Autodesk Fusion 360 part; units mm, degrees
(part 2 of 3)
  line L860 (200.8112, -803.4113) -> (192.1466, -803.4586)
  line L861 (192.1466, -803.4586) -> (192.1301, -800.4585)
  line L862 (192.1301, -800.4585) -> (183.5876, -800.5058)
  line L863 (183.5876, -800.5058) -> (183.6041, -803.5055)
  line L864 (183.6041, -803.5055) -> (174.9396, -803.5538)
  line L865 (174.9396, -803.5538) -> (174.923, -800.5538)
  line L866 (174.923, -800.5538) -> (166.3802, -800.6007)
  line L867 (166.3802, -800.6007) -> (166.3967, -803.6004)
  line L868 (166.3967, -803.6004) -> (157.7322, -803.6483)
  line L869 (157.7322, -803.6483) -> (157.7156, -800.6487)
  line L870 (157.7156, -800.6487) -> (149.1731, -800.6953)
  line L871 (149.1731, -800.6953) -> (149.1897, -803.6949)
  line L872 (149.1897, -803.6949) -> (140.5251, -803.7432)
  line L873 (140.5251, -803.7432) -> (137.5251, -803.7598)
  line L874 (137.5251, -803.7598) -> (137.5086, -800.7598)
  line L875 (137.5086, -800.7598) -> (137.5082, -800.6988)
  line L876 (137.5082, -800.6988) -> (140.5082, -800.6822)
  line L877 (140.5082, -800.6822) -> (140.5086, -800.7432)
  line L878 (140.5086, -800.7432) -> (140.4662, -793.059)
  line L879 (140.4662, -793.059) -> (137.4662, -793.0756)
  line L880 (137.4662, -793.0756) -> (137.4239, -785.3308)
  line L881 (137.4239, -785.3308) -> (140.4235, -785.3138)
  line L882 (140.4235, -785.3138) -> (140.3812, -777.691)
  line L883 (140.3812, -777.691) -> (137.3816, -777.7073)
  line L884 (137.3816, -777.7073) -> (137.3389, -769.9624)
  line L885 (137.3389, -769.9624) -> (140.3389, -769.9455)
  line L886 (140.3389, -769.9455) -> (140.2969, -762.323)
  line L887 (140.2969, -762.323) -> (137.2969, -762.3396)
  line L888 (137.2969, -762.3396) -> (137.2546, -754.5944)
  line L889 (137.2546, -754.5944) -> (140.2542, -754.5774)
  line L890 (140.2542, -754.5774) -> (140.2119, -746.9546)
  line L891 (140.2119, -746.9546) -> (137.2122, -746.9712)
  line L892 (137.2122, -746.9712) -> (137.1695, -739.226)
  line L893 (137.1695, -739.226) -> (140.1695, -739.2091)
  line L894 (140.1695, -739.2091) -> (140.1276, -731.5866)
  line L895 (140.1276, -731.5866) -> (137.1276, -731.6032)
  line L896 (137.1276, -731.6032) -> (137.0849, -723.858)
  line L897 (137.0849, -723.858) -> (140.0849, -723.8414)
  line L898 (140.0849, -723.8414) -> (140.0425, -716.2182)
  line L899 (140.0425, -716.2182) -> (137.0429, -716.2348)
  line L900 (137.0429, -716.2348) -> (137.0002, -708.49)
  line L901 (137.0002, -708.49) -> (140.0002, -708.473)
  line L902 (140.0002, -708.473) -> (139.9582, -700.8502)
  line L903 (139.9582, -700.8502) -> (136.9582, -700.8668)
  line L904 (136.9582, -700.8668) -> (136.9155, -693.1219)
  line L905 (136.9155, -693.1219) -> (139.9156, -693.105)
  line L906 (139.9156, -693.105) -> (139.8732, -685.4822)
  line L907 (139.8732, -685.4822) -> (136.8736, -685.4984)
  line L908 (136.8736, -685.4984) -> (136.8309, -677.7536)
  line L909 (136.8309, -677.7536) -> (139.8309, -677.7366)
  line L910 (139.8309, -677.7366) -> (139.7889, -670.1138)
  line L911 (139.7889, -670.1138) -> (136.7889, -670.1304)
  line L912 (136.7889, -670.1304) -> (136.7462, -662.3855)
  line L913 (136.7462, -662.3855) -> (139.7462, -662.3686)
  line L914 (139.7462, -662.3686) -> (139.7039, -654.6851)
  line L915 (139.7039, -654.6851) -> (139.7039, -654.7458)
  line L916 (139.7039, -654.7458) -> (136.7042, -654.762)
  line L917 (136.7042, -654.762) -> (136.7039, -654.7017)
  line L918 (136.7039, -654.7017) -> (136.6873, -651.7017)
  line L919 (136.6873, -651.7017) -> (139.6873, -651.6851)
  line L920 (139.6873, -651.6851) -> (148.3519, -651.6371)
  line L921 (148.3519, -651.6371) -> (148.3684, -654.6371)
  line L922 (148.3684, -654.6371) -> (156.9113, -654.5899)
  line L923 (156.9113, -654.5899) -> (156.8947, -651.5899)
  line L924 (156.8947, -651.5899) -> (165.5593, -651.5422)
  line L925 (165.5593, -651.5422) -> (165.5758, -654.5423)
  line L926 (165.5758, -654.5423) -> (174.1183, -654.4953)
  line L927 (174.1183, -654.4953) -> (174.1017, -651.4953)
  line L928 (174.1017, -651.4953) -> (182.7667, -651.4477)
  line L929 (182.7667, -651.4477) -> (182.7829, -654.4477)
  line L930 (182.7829, -654.4477) -> (191.3257, -654.4004)
  line L931 (191.3257, -654.4004) -> (191.3091, -651.4004)
  line L932 (191.3091, -651.4004) -> (199.9737, -651.3528)
  line L933 (199.9737, -651.3528) -> (199.9903, -654.3528)
  line L934 (199.9903, -654.3528) -> (208.5328, -654.3055)
  line L935 (208.5328, -654.3055) -> (208.5162, -651.3059)
  line L936 (208.5162, -651.3059) -> (217.1807, -651.2579)
  line L937 (217.1807, -651.2579) -> (217.1973, -654.2579)
  line L938 (217.1973, -654.2579) -> (225.7402, -654.211)
  line L939 (225.7402, -654.211) -> (225.7236, -651.211)
  line L940 (225.7236, -651.211) -> (234.3881, -651.163)
  line L941 (234.3881, -651.163) -> (234.4047, -654.163)
  line L942 (234.4047, -654.163) -> (242.9472, -654.1161)
  line L943 (242.9472, -654.1161) -> (242.931, -651.1161)
  line L944 (242.931, -651.1161) -> (251.5955, -651.0685)
  line L945 (251.5955, -651.0685) -> (251.6118, -654.0685)
  line L946 (251.6118, -654.0685) -> (260.1546, -654.0212)
  line L947 (260.1546, -654.0212) -> (260.138, -651.0212)
  line L948 (260.138, -651.0212) -> (268.8026, -650.9736)
  line L949 (268.8026, -650.9736) -> (268.8192, -653.9736)
  line L950 (268.8192, -653.9736) -> (277.362, -653.9263)
  line L951 (277.362, -653.9263) -> (277.3454, -650.9263)
  line L952 (277.3454, -650.9263) -> (286.01, -650.879)
  line L953 (286.01, -650.879) -> (286.0266, -653.879)
  line L954 (286.0266, -653.879) -> (294.5691, -653.8318)
  line L955 (294.5691, -653.8318) -> (294.5525, -650.8317)
  line L956 (294.5525, -650.8317) -> (303.217, -650.7841)
  line L957 (303.217, -650.7841) -> (303.2336, -653.7841)
  line L958 (303.2336, -653.7841) -> (311.7761, -653.7369)
  line L959 (311.7761, -653.7369) -> (311.7595, -650.7368)
  line L960 (311.7595, -650.7368) -> (320.4244, -650.6892)
  line L961 (320.4244, -650.6892) -> (320.441, -653.6889)
  line L962 (320.441, -653.6889) -> (328.9835, -653.6423)
  line L963 (328.9835, -653.6423) -> (328.9669, -650.6423)
  line L964 (328.9669, -650.6423) -> (337.6315, -650.5943)
  line L965 (337.6315, -650.5943) -> (337.6481, -653.5943)
  line L966 (337.6481, -653.5943) -> (346.1909, -653.5474)
  line L967 (346.1909, -653.5474) -> (346.1743, -650.5474)
  line L968 (346.1743, -650.5474) -> (354.8389, -650.4994)
  line L969 (354.8389, -650.4994) -> (354.8555, -653.4994)
  line L970 (354.8555, -653.4994) -> (363.3979, -653.4525)
  line L971 (363.3979, -653.4525) -> (363.3817, -650.4525)
  line L972 (363.3817, -650.4525) -> (372.0463, -650.4049)
  line L973 (372.0463, -650.4049) -> (372.0625, -653.4049)
  line L974 (372.0625, -653.4049) -> (380.6053, -653.3576)
  line L975 (380.6053, -653.3576) -> (380.5888, -650.3576)
  line L976 (380.5888, -650.3576) -> (389.2533, -650.31)
  line L977 (389.2533, -650.31) -> (389.2695, -653.31)
  line L978 (389.2695, -653.31) -> (397.8124, -653.2627)
  line L979 (397.8124, -653.2627) -> (397.7958, -650.2631)
  line L980 (397.7958, -650.2631) -> (406.4607, -650.2154)
  line L981 (406.4607, -650.2154) -> (406.4773, -653.2155)
  line L982 (406.4773, -653.2155) -> (415.0198, -653.1682)
  line L983 (415.0198, -653.1682) -> (415.0032, -650.1682)
  line L984 (415.0032, -650.1682) -> (423.6678, -650.1202)
  line L985 (423.6678, -650.1202) -> (423.6843, -653.1202)
  line L986 (423.6843, -653.1202) -> (432.2272, -653.0733)
  line L987 (432.2272, -653.0733) -> (432.2106, -650.0733)
  line L988 (432.2106, -650.0733) -> (440.8752, -650.0256)
  line L989 (440.8752, -650.0256) -> (440.8914, -653.0257)
  line L990 (440.8914, -653.0257) -> (449.4342, -652.9787)
  line L991 (449.4342, -652.9787) -> (449.4177, -649.9787)
  line L992 (449.4177, -649.9787) -> (458.0822, -649.9308)
  line L993 (458.0822, -649.9308) -> (458.0988, -652.9308)
  line L994 (458.0988, -652.9308) -> (466.6416, -652.8838)
  line L995 (466.6416, -652.8838) -> (466.6251, -649.8838)
  line L996 (466.6251, -649.8838) -> (475.2893, -649.8362)
  line L997 (475.2893, -649.8362) -> (475.3058, -652.8359)
  line L998 (475.3058, -652.8359) -> (483.8487, -652.789)
  line L999 (483.8487, -652.789) -> (483.8321, -649.7889)
  line L1000 (483.8321, -649.7889) -> (492.497, -649.7413)
  line L1001 (492.497, -649.7413) -> (492.5132, -652.7413)
  line L1002 (492.5132, -652.7413) -> (501.0557, -652.6941)
  line L1003 (501.0557, -652.6941) -> (501.0391, -649.694)
  line L1004 (501.0391, -649.694) -> (509.7041, -649.6464)
  line L1005 (509.7041, -649.6464) -> (509.7206, -652.6464)
  line L1006 (509.7206, -652.6464) -> (518.2635, -652.5995)
  line L1007 (518.2635, -652.5995) -> (518.2469, -649.5995)
  line L1008 (518.2469, -649.5995) -> (526.9111, -649.5515)
  line L1009 (526.9111, -649.5515) -> (526.9277, -652.5515)
  line L1010 (526.9277, -652.5515) -> (535.4705, -652.5046)
  line L1011 (535.4705, -652.5046) -> (535.4539, -649.5046)
  line L1012 (535.4539, -649.5046) -> (544.1185, -649.4566)
  line L1013 (544.1185, -649.4566) -> (544.1351, -652.4566)
  line L1014 (544.1351, -652.4566) -> (552.6776, -652.4097)
  line L1015 (552.6776, -652.4097) -> (552.6613, -649.4101)
  line L1016 (552.6613, -649.4101) -> (561.3255, -649.3621)
  line L1017 (561.3255, -649.3621) -> (561.3421, -652.3621)
  line L1018 (561.3421, -652.3621) -> (569.885, -652.3152)
  line L1019 (569.885, -652.3152) -> (569.8684, -649.3152)
  line L1020 (569.8684, -649.3152) -> (578.5329, -649.2672)
  line L1021 (578.5329, -649.2672) -> (578.5495, -652.2672)
  line L1022 (578.5495, -652.2672) -> (587.092, -652.2199)
  line L1023 (587.092, -652.2199) -> (587.0754, -649.2199)
  line L1024 (587.0754, -649.2199) -> (595.7403, -649.1726)
  line L1025 (595.7403, -649.1726) -> (598.7404, -649.1561)
  line L1026 (598.7404, -649.1561) -> (598.7569, -652.1561)
  line L1027 (598.7569, -652.1561) -> (598.7573, -652.2171)
  line L1028 (598.7573, -652.2171) -> (595.7573, -652.2333)
  line L1029 (3.1447, -620.2227) -> (3.1447, -628.8876)
  line L1030 (3.1447, -628.8876) -> (6.1443, -628.8876)
  line L1031 (6.1443, -620.2227) -> (3.1447, -620.2227)
  line L1032 (3.1447, -603.0153) -> (3.1447, -611.6799)
  line L1033 (3.1447, -611.6799) -> (6.1443, -611.6799)
  line L1034 (6.1443, -603.0153) -> (3.1447, -603.0153)
  line L1035 (3.1447, -585.8079) -> (3.1447, -594.4725)
  line L1036 (3.1447, -594.4725) -> (6.1443, -594.4725)
  line L1037 (6.1443, -585.8079) -> (3.1447, -585.8079)
  line L1038 (3.1447, -568.6002) -> (3.1447, -577.2651)
  line L1039 (3.1447, -577.2651) -> (6.1443, -577.2651)
  line L1040 (6.1443, -568.6002) -> (3.1447, -568.6002)
  line L1041 (3.1447, -551.3928) -> (3.1447, -560.0573)
  line L1042 (3.1447, -560.0573) -> (6.1443, -560.0573)
  line L1043 (6.1443, -551.3928) -> (3.1447, -551.3928)
  line L1044 (3.1447, -534.185) -> (3.1447, -542.8499)
  line L1045 (3.1447, -542.8499) -> (6.1443, -542.8499)
  line L1046 (6.1443, -534.185) -> (3.1447, -534.185)
  line L1047 (3.1447, -516.9776) -> (3.1447, -525.6425)
  line L1048 (3.1447, -525.6425) -> (6.1443, -525.6425)
  line L1049 (6.1443, -516.9776) -> (3.1447, -516.9776)
  line L1050 (3.1447, -499.7702) -> (3.1447, -508.4348)
  line L1051 (3.1447, -508.4348) -> (6.1443, -508.4348)
  line L1052 (6.1443, -499.7702) -> (3.1447, -499.7702)
  line L1053 (3.1447, -482.5625) -> (3.1447, -491.2274)
  line L1054 (3.1447, -491.2274) -> (6.1443, -491.2274)
  line L1055 (6.1443, -482.5625) -> (3.1447, -482.5625)
  line L1056 (3.1447, -465.3551) -> (3.1447, -474.02)
  line L1057 (3.1447, -474.02) -> (6.1443, -474.02)
  line L1058 (6.1443, -465.3551) -> (3.1447, -465.3551)
  line L1059 (3.1447, -448.1477) -> (3.1447, -456.8122)
  line L1060 (3.1447, -456.8122) -> (6.1443, -456.8122)
  line L1061 (6.1443, -448.1477) -> (3.1447, -448.1477)
  line L1062 (3.1447, -430.9403) -> (3.1447, -439.6048)
  line L1063 (3.1447, -439.6048) -> (6.1443, -439.6048)
  line L1064 (6.1443, -430.9403) -> (3.1447, -430.9403)
  line L1065 (3.1447, -413.7329) -> (3.1447, -422.3974)
  line L1066 (3.1447, -422.3974) -> (6.1443, -422.3974)
  line L1067 (6.1443, -413.7329) -> (3.1447, -413.7329)
  line L1068 (3.1447, -396.5255) -> (3.1447, -405.1897)
  line L1069 (3.1447, -405.1897) -> (6.1443, -405.1897)
  line L1070 (6.1443, -396.5255) -> (3.1447, -396.5255)
  line L1071 (3.1447, -379.3177) -> (3.1447, -387.9826)
  line L1072 (3.1447, -387.9826) -> (6.1443, -387.9826)
  line L1073 (6.1443, -379.3177) -> (3.1447, -379.3177)
  line L1074 (3.1447, -362.1103) -> (3.1447, -370.7752)
  line L1075 (3.1447, -370.7752) -> (6.1443, -370.7752)
  line L1076 (6.1443, -362.1103) -> (3.1447, -362.1103)
  line L1077 (3.1447, -344.9029) -> (3.1447, -353.5675)
  line L1078 (3.1447, -353.5675) -> (6.1443, -353.5675)
  line L1079 (6.1443, -344.9029) -> (3.1447, -344.9029)
  line L1080 (3.1447, -327.6952) -> (3.1447, -336.3601)
  line L1081 (3.1447, -336.3601) -> (6.1443, -336.3601)
  line L1082 (6.1443, -327.6952) -> (3.1447, -327.6952)
  line L1083 (3.1447, -310.4878) -> (3.1447, -319.1527)
  line L1084 (3.1447, -319.1527) -> (6.1443, -319.1527)
  line L1085 (6.1443, -310.4878) -> (3.1447, -310.4878)
  line L1086 (3.1447, -293.2804) -> (3.1447, -301.9449)
  line L1087 (3.1447, -301.9449) -> (6.1443, -301.9449)
  line L1088 (6.1443, -293.2804) -> (3.1447, -293.2804)
  line L1089 (3.1447, -276.0726) -> (3.1447, -284.7375)
  line L1090 (3.1447, -284.7375) -> (6.1443, -284.7375)
  line L1091 (6.1443, -276.0726) -> (3.1447, -276.0726)
  line L1092 (3.1447, -258.8652) -> (3.1447, -267.5298)
  line L1093 (3.1447, -267.5298) -> (6.1443, -267.5298)
  line L1094 (6.1443, -258.8652) -> (3.1447, -258.8652)
  line L1095 (3.1447, -241.6578) -> (3.1447, -250.3224)
  line L1096 (3.1447, -250.3224) -> (6.1443, -250.3224)
  line L1097 (6.1443, -241.6578) -> (3.1447, -241.6578)
  line L1098 (3.1447, -224.4501) -> (3.1447, -233.115)
  line L1099 (3.1447, -233.115) -> (6.1443, -233.115)
  line L1100 (6.1443, -224.4501) -> (3.1447, -224.4501)
  line L1101 (3.1447, -207.2427) -> (3.1447, -215.9072)
  line L1102 (3.1447, -215.9072) -> (6.1443, -215.9072)
  line L1103 (6.1443, -207.2427) -> (3.1447, -207.2427)
  line L1104 (3.1447, -190.0353) -> (3.1447, -198.6998)
  line L1105 (3.1447, -198.6998) -> (6.1443, -198.6998)
  line L1106 (6.1443, -190.0353) -> (3.1447, -190.0353)
  line L1107 (6.1443, -628.8876) -> (6.1443, -637.4911)
  line L1108 (6.1443, -637.4911) -> (14.811, -637.4911)
  line L1109 (6.1443, -611.6799) -> (6.1443, -620.2227)
  line L1110 (6.1443, -594.4725) -> (6.1443, -603.0153)
  line L1111 (6.1443, -577.2651) -> (6.1443, -585.8079)
  line L1112 (6.1443, -560.0573) -> (6.1443, -568.6002)
  line L1113 (6.1443, -542.8499) -> (6.1443, -551.3928)
  line L1114 (6.1443, -525.6425) -> (6.1443, -534.185)
  line L1115 (6.1443, -508.4348) -> (6.1443, -516.9776)
  line L1116 (6.1443, -491.2274) -> (6.1443, -499.7702)
  line L1117 (6.1443, -474.02) -> (6.1443, -482.5625)
  line L1118 (6.1443, -456.8122) -> (6.1443, -465.3551)
  line L1119 (6.1443, -439.6048) -> (6.1443, -448.1477)
  line L1120 (6.1443, -422.3974) -> (6.1443, -430.9403)
  line L1121 (6.1443, -405.1897) -> (6.1443, -413.7329)
  line L1122 (6.1443, -387.9826) -> (6.1443, -396.5255)
  line L1123 (6.1443, -370.7752) -> (6.1443, -379.3177)
  line L1124 (6.1443, -353.5675) -> (6.1443, -362.1103)
  line L1125 (6.1443, -336.3601) -> (6.1443, -344.9029)
  line L1126 (6.1443, -319.1527) -> (6.1443, -327.6952)
  line L1127 (6.1443, -301.9449) -> (6.1443, -310.4878)
  line L1128 (6.1443, -284.7375) -> (6.1443, -293.2804)
  line L1129 (6.1443, -267.5298) -> (6.1443, -276.0726)
  line L1130 (6.1443, -250.3224) -> (6.1443, -258.8652)
  line L1131 (6.1443, -233.115) -> (6.1443, -241.6578)
  line L1132 (6.1443, -215.9072) -> (6.1443, -224.4501)
  line L1133 (6.1443, -198.6998) -> (6.1443, -207.2427)
  line L1134 (6.1443, -181.4314) -> (6.1443, -190.0353)
  line L1135 (14.811, -181.4314) -> (6.1443, -181.4314)
  line L1136 (14.811, -637.4911) -> (14.811, -640.4911)
  line L1137 (14.811, -640.4911) -> (23.539, -640.4911)
  line L1138 (14.811, -178.4314) -> (14.811, -181.4314)
  line L1139 (23.5387, -178.4314) -> (14.811, -178.4314)
  line L1140 (23.5387, -640.4911) -> (23.5387, -637.4911)
  line L1141 (23.5387, -637.4911) -> (32.1443, -637.4911)
  line L1142 (23.5387, -181.4314) -> (23.5387, -178.4314)
  line L1143 (32.1443, -181.4314) -> (23.5387, -181.4314)
  line L1144 (32.1443, -637.4911) -> (32.1443, -640.4911)
  line L1145 (32.1443, -640.4911) -> (40.872, -640.4911)
  line L1146 (32.1443, -178.4314) -> (32.1443, -181.4314)
  line L1147 (40.872, -178.4314) -> (32.1443, -178.4314)
  line L1148 (40.872, -640.4911) -> (40.872, -637.4911)
  line L1149 (40.872, -637.4911) -> (49.4777, -637.4911)
  line L1150 (40.872, -181.4314) -> (40.872, -178.4314)
  line L1151 (49.4777, -181.4314) -> (40.872, -181.4314)
  line L1152 (49.4777, -637.4911) -> (49.4777, -640.4911)
  line L1153 (49.4777, -640.4911) -> (58.2054, -640.4911)
  line L1154 (49.4777, -178.4314) -> (49.4777, -181.4314)
  line L1155 (58.2054, -178.4314) -> (49.4773, -178.4314)
  line L1156 (58.2054, -640.4911) -> (58.2054, -637.4911)
  line L1157 (58.2054, -637.4911) -> (66.8114, -637.4911)
  line L1158 (58.2054, -181.4314) -> (58.2054, -178.4314)
  line L1159 (66.811, -181.4314) -> (58.205, -181.4314)
  line L1160 (66.811, -637.4911) -> (66.811, -640.4911)
  line L1161 (66.811, -640.4911) -> (75.5387, -640.4911)
  line L1162 (66.811, -178.4314) -> (66.811, -181.4314)
  line L1163 (75.5387, -178.4314) -> (66.811, -178.4314)
  line L1164 (75.5387, -640.4911) -> (75.5387, -637.4911)
  line L1165 (75.5387, -637.4911) -> (84.1443, -637.4911)
  line L1166 (75.5387, -181.4314) -> (75.5387, -178.4314)
  line L1167 (84.1443, -181.4314) -> (75.5387, -181.4314)
  line L1168 (84.1443, -637.4911) -> (84.1443, -640.4911)
  line L1169 (84.1443, -640.4911) -> (92.872, -640.4911)
  line L1170 (84.1443, -178.4314) -> (84.1443, -181.4314)
  line L1171 (92.872, -178.4314) -> (84.1443, -178.4314)
  line L1172 (92.872, -640.4911) -> (92.872, -637.4911)
  line L1173 (92.872, -637.4911) -> (101.4777, -637.4911)
  line L1174 (92.872, -181.4314) -> (92.872, -178.4314)
  line L1175 (101.4777, -181.4314) -> (92.872, -181.4314)
  line L1176 (101.4777, -637.4911) -> (101.4777, -640.4911)
  line L1177 (101.4777, -640.4911) -> (110.2054, -640.4911)
  line L1178 (101.4777, -178.4314) -> (101.4777, -181.4314)
  line L1179 (110.2054, -178.4314) -> (101.4773, -178.4314)
  line L1180 (110.2054, -640.4911) -> (110.2054, -637.4911)
  line L1181 (110.2054, -637.4911) -> (118.811, -637.4911)
  line L1182 (110.2054, -181.4314) -> (110.2054, -178.4314)
  line L1183 (118.811, -181.4314) -> (110.2054, -181.4314)
  line L1184 (118.811, -637.4911) -> (118.811, -640.4911)
  line L1185 (118.811, -640.4911) -> (127.5384, -640.4911)
  line L1186 (118.811, -178.4314) -> (118.811, -181.4314)
  line L1187 (127.5384, -178.4314) -> (118.8107, -178.4314)
  line L1188 (127.5384, -640.4911) -> (127.5384, -637.4911)
  line L1189 (127.5384, -637.4911) -> (136.144, -637.4911)
  line L1190 (127.5384, -181.4314) -> (127.5384, -178.4314)
  line L1191 (136.144, -181.4314) -> (127.5384, -181.4314)
  line L1192 (136.144, -637.4911) -> (136.144, -640.4911)
  line L1193 (136.144, -640.4911) -> (144.8717, -640.4911)
  line L1194 (136.144, -178.4314) -> (136.144, -181.4314)
  line L1195 (144.8717, -178.4314) -> (136.144, -178.4314)
  line L1196 (144.8717, -640.4911) -> (144.8717, -637.4911)
  line L1197 (144.8717, -637.4911) -> (153.4774, -637.4911)
  line L1198 (144.8717, -181.4314) -> (144.8717, -178.4314)
  line L1199 (153.4774, -181.4314) -> (144.8717, -181.4314)
  line L1200 (153.4774, -637.4911) -> (153.4774, -640.4911)
  line L1201 (153.4774, -640.4911) -> (162.2051, -640.4911)
  line L1202 (153.4774, -178.4314) -> (153.4774, -181.4314)
  line L1203 (162.2051, -178.4314) -> (153.4774, -178.4314)
  line L1204 (162.2051, -640.4911) -> (162.2051, -637.4911)
  line L1205 (162.2051, -637.4911) -> (170.811, -637.4911)
  line L1206 (162.2051, -181.4314) -> (162.2051, -178.4314)
  line L1207 (170.8107, -181.4314) -> (162.2047, -181.4314)
  line L1208 (170.8107, -637.4911) -> (170.8107, -640.4911)
  line L1209 (170.8107, -640.4911) -> (179.5384, -640.4911)
  line L1210 (170.8107, -178.4314) -> (170.8107, -181.4314)
  line L1211 (179.5384, -178.4314) -> (170.8107, -178.4314)
  line L1212 (179.5384, -640.4911) -> (179.5384, -637.4911)
  line L1213 (179.5384, -637.4911) -> (188.1444, -637.4911)
  line L1214 (179.5384, -181.4314) -> (179.5384, -178.4314)
  line L1215 (188.144, -181.4314) -> (179.538, -181.4314)
  line L1216 (188.144, -637.4911) -> (188.144, -640.4911)
  line L1217 (188.144, -640.4911) -> (196.8717, -640.4911)
  line L1218 (188.144, -178.4314) -> (188.144, -181.4314)
  line L1219 (196.8717, -178.4314) -> (188.144, -178.4314)
  line L1220 (196.8717, -640.4911) -> (196.8717, -637.4911)
  line L1221 (196.8717, -637.4911) -> (205.4774, -637.4911)
  line L1222 (196.8717, -181.4314) -> (196.8717, -178.4314)
  line L1223 (205.4774, -181.4314) -> (196.8717, -181.4314)
  line L1224 (205.4774, -637.4911) -> (205.4774, -640.4911)
  line L1225 (205.4774, -640.4911) -> (214.2051, -640.4911)
  line L1226 (205.4774, -178.4314) -> (205.4774, -181.4314)
  line L1227 (214.2051, -178.4314) -> (205.4774, -178.4314)
  line L1228 (214.2051, -640.4911) -> (214.2051, -637.4911)
  line L1229 (214.2051, -637.4911) -> (222.8107, -637.4911)
  line L1230 (214.2051, -181.4314) -> (214.2051, -178.4314)
  line L1231 (222.8107, -181.4314) -> (214.2051, -181.4314)
  line L1232 (222.8107, -637.4911) -> (222.8107, -640.4911)
  line L1233 (222.8107, -640.4911) -> (231.5384, -640.4911)
  line L1234 (222.8107, -178.4314) -> (222.8107, -181.4314)
  line L1235 (231.5384, -178.4314) -> (222.8107, -178.4314)
  line L1236 (231.5384, -640.4911) -> (231.5384, -637.4911)
  line L1237 (231.5384, -637.4911) -> (240.1441, -637.4911)
  line L1238 (231.5384, -181.4314) -> (231.5384, -178.4314)
  line L1239 (240.1441, -181.4314) -> (231.5384, -181.4314)
  line L1240 (240.1441, -637.4911) -> (240.1441, -640.4911)
  line L1241 (240.1441, -640.4911) -> (248.8718, -640.4911)
  line L1242 (240.1441, -178.4314) -> (240.1441, -181.4314)
  line L1243 (248.8714, -178.4314) -> (240.1441, -178.4314)
  line L1244 (248.8714, -640.4911) -> (248.8714, -637.4911)
  line L1245 (248.8714, -637.4911) -> (257.477, -637.4911)
  line L1246 (248.8714, -181.4314) -> (248.8714, -178.4314)
  line L1247 (257.477, -181.4314) -> (248.8714, -181.4314)
  line L1248 (257.477, -637.4911) -> (257.477, -640.4911)
  line L1249 (257.477, -640.4911) -> (266.2051, -640.4911)
  line L1250 (257.477, -178.4314) -> (257.477, -181.4314)
  line L1251 (266.2047, -178.4314) -> (257.477, -178.4314)
  line L1252 (266.2047, -640.4911) -> (266.2047, -637.4911)
  line L1253 (266.2047, -637.4911) -> (274.8104, -637.4911)
  line L1254 (266.2047, -181.4314) -> (266.2047, -178.4314)
  line L1255 (274.8104, -181.4314) -> (266.2047, -181.4314)
  line L1256 (274.8104, -637.4911) -> (274.8104, -640.4911)
  line L1257 (274.8104, -640.4911) -> (283.5381, -640.4911)
  line L1258 (274.8104, -178.4314) -> (274.8104, -181.4314)
  line L1259 (283.5381, -178.4314) -> (274.8104, -178.4314)
  line L1260 (283.5381, -640.4911) -> (283.5381, -637.4911)
  line L1261 (283.5381, -637.4911) -> (292.2048, -637.4911)
  line L1262 (283.5381, -181.4314) -> (283.5381, -178.4314)
  line L1263 (292.2048, -181.4314) -> (283.5381, -181.4314)
  line L1264 (292.2048, -637.4911) -> (292.2048, -628.8873)
  line L1265 (292.2048, -628.8876) -> (295.2048, -628.8876)
  line L1266 (292.2048, -620.2227) -> (292.2048, -611.6799)
  line L1267 (295.2048, -620.2227) -> (292.2048, -620.2227)
  line L1268 (292.2048, -611.6799) -> (295.2048, -611.6799)
  line L1269 (292.2048, -603.0153) -> (292.2048, -594.4725)
  line L1270 (295.2048, -603.0153) -> (292.2048, -603.0153)
  line L1271 (292.2048, -594.4725) -> (295.2048, -594.4725)
  line L1272 (292.2048, -585.8079) -> (292.2048, -577.2651)
  line L1273 (295.2048, -585.8079) -> (292.2048, -585.8079)
  line L1274 (292.2048, -577.2651) -> (295.2048, -577.2651)
  line L1275 (292.2048, -568.6002) -> (292.2048, -560.0573)
  line L1276 (295.2048, -568.6002) -> (292.2048, -568.6002)
  line L1277 (292.2048, -560.0573) -> (295.2048, -560.0573)
  line L1278 (292.2048, -551.3928) -> (292.2048, -542.8499)
  line L1279 (295.2048, -551.3928) -> (292.2048, -551.3928)
  line L1280 (292.2048, -542.8499) -> (295.2048, -542.8499)
  line L1281 (292.2048, -534.185) -> (292.2048, -525.6425)
  line L1282 (295.2048, -534.185) -> (292.2048, -534.185)
  line L1283 (292.2048, -525.6425) -> (295.2048, -525.6425)
  line L1284 (292.2048, -516.9776) -> (292.2048, -508.4348)
  line L1285 (295.2048, -516.9776) -> (292.2048, -516.9776)
  line L1286 (292.2048, -508.4348) -> (295.2048, -508.4348)
  line L1287 (292.2048, -499.7702) -> (292.2048, -491.2274)
  line L1288 (295.2048, -499.7702) -> (292.2048, -499.7702)
  line L1289 (292.2048, -491.2274) -> (295.2048, -491.2274)
  line L1290 (292.2048, -482.5625) -> (292.2048, -474.02)
  line L1291 (295.2048, -482.5625) -> (292.2048, -482.5625)
  line L1292 (292.2048, -474.02) -> (295.2048, -474.02)
  line L1293 (292.2048, -465.3551) -> (292.2048, -456.8122)
  line L1294 (295.2048, -465.3551) -> (292.2048, -465.3551)
  line L1295 (292.2048, -456.8122) -> (295.2048, -456.8122)
  line L1296 (292.2048, -448.1477) -> (292.2048, -439.6048)
  line L1297 (295.2048, -448.1477) -> (292.2048, -448.1477)
  line L1298 (292.2048, -439.6048) -> (295.2048, -439.6048)
  line L1299 (292.2048, -430.9403) -> (292.2048, -422.3974)
  line L1300 (295.2048, -430.9403) -> (292.2048, -430.9403)
  line L1301 (292.2048, -422.3974) -> (295.2048, -422.3974)
  line L1302 (292.2048, -413.7329) -> (292.2048, -405.1897)
  line L1303 (295.2048, -413.7329) -> (292.2048, -413.7329)
  line L1304 (292.2048, -405.1897) -> (295.2048, -405.1897)
  line L1305 (292.2048, -396.5255) -> (292.2048, -387.9823)
  line L1306 (295.2048, -396.5255) -> (292.2048, -396.5255)
  line L1307 (292.2048, -387.9826) -> (295.2048, -387.9826)
  line L1308 (292.2048, -379.3177) -> (292.2048, -370.7749)
  line L1309 (295.2048, -379.3177) -> (292.2048, -379.3177)
  line L1310 (292.2048, -370.7752) -> (295.2048, -370.7752)
  line L1311 (292.2048, -362.1103) -> (292.2048, -353.5675)
  line L1312 (295.2048, -362.1103) -> (292.2048, -362.1103)
  line L1313 (292.2048, -353.5675) -> (295.2048, -353.5675)
  line L1314 (292.2048, -344.9029) -> (292.2048, -336.3597)
  line L1315 (295.2048, -344.9029) -> (292.2048, -344.9029)
  line L1316 (292.2048, -336.3601) -> (295.2048, -336.3601)
  line L1317 (292.2048, -327.6952) -> (292.2048, -319.1523)
  line L1318 (295.2048, -327.6952) -> (292.2048, -327.6952)
  line L1319 (292.2048, -319.1527) -> (295.2048, -319.1527)
  line L1320 (292.2048, -310.4878) -> (292.2048, -301.9449)
  line L1321 (295.2048, -310.4878) -> (292.2048, -310.4878)
  line L1322 (292.2048, -301.9449) -> (295.2048, -301.9449)
  line L1323 (292.2048, -293.2804) -> (292.2048, -284.7372)
  line L1324 (295.2048, -293.2804) -> (292.2048, -293.2804)
  line L1325 (292.2048, -284.7375) -> (295.2048, -284.7375)
  line L1326 (292.2048, -276.0726) -> (292.2048, -267.5298)
  line L1327 (295.2048, -276.0726) -> (292.2048, -276.0726)
  line L1328 (292.2048, -267.5298) -> (295.2048, -267.5298)
  line L1329 (292.2048, -258.8652) -> (292.2048, -250.3224)
  line L1330 (295.2048, -258.8652) -> (292.2048, -258.8652)
  line L1331 (292.2048, -250.3224) -> (295.2048, -250.3224)
  line L1332 (292.2048, -241.6578) -> (292.2048, -233.1146)
  line L1333 (295.2048, -241.6578) -> (292.2048, -241.6578)
  line L1334 (292.2048, -233.115) -> (295.2048, -233.115)
  line L1335 (292.2048, -224.4501) -> (292.2048, -215.9072)
  line L1336 (295.2048, -224.4501) -> (292.2048, -224.4501)
  line L1337 (292.2048, -215.9072) -> (295.2048, -215.9072)
  line L1338 (292.2048, -207.2427) -> (292.2048, -198.6998)
  line L1339 (295.2048, -207.2427) -> (292.2048, -207.2427)
  line L1340 (292.2048, -198.6998) -> (295.2048, -198.6998)
  line L1341 (292.2048, -190.0353) -> (292.2048, -181.431)
  line L1342 (295.2048, -190.0353) -> (292.2048, -190.0353)
  line L1343 (295.2048, -628.8876) -> (295.2048, -620.2224)
  line L1344 (295.2048, -611.6799) -> (295.2048, -603.015)
  line L1345 (295.2048, -594.4725) -> (295.2048, -585.8076)
  line L1346 (295.2048, -577.2651) -> (295.2048, -568.5998)
  line L1347 (295.2048, -560.0573) -> (295.2048, -551.3924)
  line L1348 (295.2048, -542.8499) -> (295.2048, -534.185)
  line L1349 (295.2048, -525.6425) -> (295.2048, -516.9773)
  line L1350 (295.2048, -508.4348) -> (295.2048, -499.7699)
  line L1351 (295.2048, -491.2274) -> (295.2048, -482.5621)
  line L1352 (295.2048, -474.02) -> (295.2048, -465.3547)
  line L1353 (295.2048, -456.8122) -> (295.2048, -448.1473)
  line L1354 (295.2048, -439.6048) -> (295.2048, -430.9399)
  line L1355 (295.2048, -422.3974) -> (295.2048, -413.7325)
  line L1356 (295.2048, -405.1897) -> (295.2048, -396.5251)
  line L1357 (295.2048, -387.9826) -> (295.2048, -379.3177)
  line L1358 (295.2048, -370.7752) -> (295.2048, -362.1103)
  line L1359 (295.2048, -353.5675) -> (295.2048, -344.9026)
  line L1360 (295.2048, -336.3601) -> (295.2048, -327.6952)
  line L1361 (295.2048, -319.1527) -> (295.2048, -310.4878)
  line L1362 (295.2048, -301.9449) -> (295.2048, -293.28)
  line L1363 (295.2048, -284.7375) -> (295.2048, -276.0726)
  line L1364 (295.2048, -267.5298) -> (295.2048, -258.8649)
  line L1365 (295.2048, -250.3224) -> (295.2048, -241.6575)
  line L1366 (295.2048, -233.115) -> (295.2048, -224.4501)
  line L1367 (295.2048, -215.9072) -> (295.2048, -207.2423)
  line L1368 (295.2048, -198.6998) -> (295.2048, -190.0349)
  line L1369 (452.2233, -620.2227) -> (452.2233, -628.8876)
  line L1370 (452.2233, -628.8876) -> (455.2233, -628.8876)
  line L1371 (455.2233, -620.2227) -> (452.2233, -620.2227)
  line L1372 (452.2233, -603.0153) -> (452.2233, -611.6799)
  line L1373 (452.2233, -611.6799) -> (455.2233, -611.6799)
  line L1374 (455.2233, -603.0153) -> (452.2233, -603.0153)
  line L1375 (452.2233, -585.8079) -> (452.2233, -594.4725)
  line L1376 (452.2233, -594.4725) -> (455.2233, -594.4725)
  line L1377 (455.2233, -585.8079) -> (452.2233, -585.8079)
  line L1378 (452.2233, -568.6002) -> (452.2233, -577.2651)
  line L1379 (452.2233, -577.2651) -> (455.2233, -577.2651)
  line L1380 (455.2233, -568.6002) -> (452.2233, -568.6002)
  line L1381 (452.2233, -551.3928) -> (452.2233, -560.0573)
  line L1382 (452.2233, -560.0573) -> (455.2233, -560.0573)
  line L1383 (455.2233, -551.3928) -> (452.2233, -551.3928)
  line L1384 (452.2233, -534.185) -> (452.2233, -542.8499)
  line L1385 (452.2233, -542.8499) -> (455.2233, -542.8499)
  line L1386 (455.2233, -534.185) -> (452.2233, -534.185)
  line L1387 (452.2233, -516.9776) -> (452.2233, -525.6425)
  line L1388 (452.2233, -525.6425) -> (455.2233, -525.6425)
  line L1389 (455.2233, -516.9776) -> (452.2233, -516.9776)
  line L1390 (452.2233, -499.7702) -> (452.2233, -508.4348)
  line L1391 (452.2233, -508.4348) -> (455.2233, -508.4348)
  line L1392 (455.2233, -499.7702) -> (452.2233, -499.7702)
  line L1393 (452.2233, -482.5625) -> (452.2233, -491.2274)
  line L1394 (452.2233, -491.2274) -> (455.2233, -491.2274)
  line L1395 (455.2233, -482.5625) -> (452.2233, -482.5625)
  line L1396 (452.2233, -465.3551) -> (452.2233, -474.02)
  line L1397 (452.2233, -474.02) -> (455.2233, -474.02)
  line L1398 (455.2233, -465.3551) -> (452.2233, -465.3551)
  line L1399 (452.2233, -448.1477) -> (452.2233, -456.8122)
  line L1400 (452.2233, -456.8122) -> (455.2233, -456.8122)
  line L1401 (455.2233, -448.1477) -> (452.2233, -448.1477)
  line L1402 (452.2233, -430.9403) -> (452.2233, -439.6048)
  line L1403 (452.2233, -439.6048) -> (455.2233, -439.6048)
  line L1404 (455.2233, -430.9403) -> (452.2233, -430.9403)
  line L1405 (452.2233, -413.7329) -> (452.2233, -422.3974)
  line L1406 (452.2233, -422.3974) -> (455.2233, -422.3974)
  line L1407 (455.2233, -413.7329) -> (452.2233, -413.7329)
  line L1408 (452.2233, -396.5255) -> (452.2233, -405.1897)
  line L1409 (452.2233, -405.1897) -> (455.2233, -405.1897)
  line L1410 (455.2233, -396.5255) -> (452.2233, -396.5255)
  line L1411 (452.2233, -379.3177) -> (452.2233, -387.9826)
  line L1412 (452.2233, -387.9826) -> (455.2233, -387.9826)
  line L1413 (455.2233, -379.3177) -> (452.2233, -379.3177)
  line L1414 (452.2233, -362.1103) -> (452.2233, -370.7752)
  line L1415 (452.2233, -370.7752) -> (455.2233, -370.7752)
  line L1416 (455.2233, -362.1103) -> (452.2233, -362.1103)
  line L1417 (452.2233, -344.9029) -> (452.2233, -353.5675)
  line L1418 (452.2233, -353.5675) -> (455.2233, -353.5675)
  line L1419 (455.2233, -344.9029) -> (452.2233, -344.9029)
  line L1420 (452.2233, -327.6952) -> (452.2233, -336.3601)
  line L1421 (452.2233, -336.3601) -> (455.2233, -336.3601)
  line L1422 (455.2233, -327.6952) -> (452.2233, -327.6952)
  line L1423 (452.2233, -310.4878) -> (452.2233, -319.1527)
  line L1424 (452.2233, -319.1527) -> (455.2233, -319.1527)
  line L1425 (455.2233, -310.4878) -> (452.2233, -310.4878)
  line L1426 (452.2233, -293.2804) -> (452.2233, -301.9449)
  line L1427 (452.2233, -301.9449) -> (455.2233, -301.9449)
  line L1428 (455.2233, -293.2804) -> (452.2233, -293.2804)
  line L1429 (452.2233, -276.0726) -> (452.2233, -284.7375)
  line L1430 (452.2233, -284.7375) -> (455.2233, -284.7375)
  line L1431 (455.2233, -276.0726) -> (452.2233, -276.0726)
  line L1432 (452.2233, -258.8652) -> (452.2233, -267.5298)
  line L1433 (452.2233, -267.5298) -> (455.2233, -267.5298)
  line L1434 (455.2233, -258.8652) -> (452.2233, -258.8652)
  line L1435 (452.2233, -241.6578) -> (452.2233, -250.3224)
  line L1436 (452.2233, -250.3224) -> (455.2233, -250.3224)
  line L1437 (455.2233, -241.6578) -> (452.2233, -241.6578)
  line L1438 (452.2233, -224.4501) -> (452.2233, -233.115)
  line L1439 (452.2233, -233.115) -> (455.2233, -233.115)
  line L1440 (455.2233, -224.4501) -> (452.2233, -224.4501)
  line L1441 (452.2233, -207.2427) -> (452.2233, -215.9072)
  line L1442 (452.2233, -215.9072) -> (455.2233, -215.9072)
  line L1443 (455.2233, -207.2427) -> (452.2233, -207.2427)
  line L1444 (452.2233, -190.0353) -> (452.2233, -198.6998)
  line L1445 (452.2233, -198.6998) -> (455.2233, -198.6998)
  line L1446 (455.2233, -190.0353) -> (452.2233, -190.0353)
  line L1447 (463.89, -181.4314) -> (455.2233, -181.4314)
  line L1448 (455.2233, -628.8876) -> (455.2233, -637.4911)
  line L1449 (455.2233, -637.4911) -> (463.89, -637.4911)
  line L1450 (455.2233, -611.6799) -> (455.2233, -620.2227)
  line L1451 (455.2233, -594.4725) -> (455.2233, -603.0153)
  line L1452 (455.2233, -577.2651) -> (455.2233, -585.8079)
  line L1453 (455.2233, -560.0573) -> (455.2233, -568.6002)
  line L1454 (455.2233, -542.8499) -> (455.2233, -551.3928)
  line L1455 (455.2233, -525.6425) -> (455.2233, -534.185)
  line L1456 (455.2233, -508.4348) -> (455.2233, -516.9776)
  line L1457 (455.2233, -491.2274) -> (455.2233, -499.7702)
  line L1458 (455.2233, -474.02) -> (455.2233, -482.5625)
  line L1459 (455.2233, -456.8122) -> (455.2233, -465.3551)
  line L1460 (455.2233, -439.6048) -> (455.2233, -448.1477)
  line L1461 (455.2233, -422.3974) -> (455.2233, -430.9403)
  line L1462 (455.2233, -405.1897) -> (455.2233, -413.7329)
  line L1463 (455.2233, -387.9826) -> (455.2233, -396.5255)
  line L1464 (455.2233, -370.7752) -> (455.2233, -379.3177)
  line L1465 (455.2233, -353.5675) -> (455.2233, -362.1103)
  line L1466 (455.2233, -336.3601) -> (455.2233, -344.9029)
  line L1467 (455.2233, -319.1527) -> (455.2233, -327.6952)
  line L1468 (455.2233, -301.9449) -> (455.2233, -310.4878)
  line L1469 (455.2233, -284.7375) -> (455.2233, -293.2804)
  line L1470 (455.2233, -267.5298) -> (455.2233, -276.0726)
  line L1471 (455.2233, -250.3224) -> (455.2233, -258.8652)
  line L1472 (455.2233, -233.115) -> (455.2233, -241.6578)
  line L1473 (455.2233, -215.9072) -> (455.2233, -224.4501)
  line L1474 (455.2233, -198.6998) -> (455.2233, -207.2427)
  line L1475 (455.2233, -181.4314) -> (455.2233, -190.0353)
  line L1476 (463.89, -178.4314) -> (463.89, -181.4314)
  line L1477 (472.6177, -178.4314) -> (463.89, -178.4314)
  line L1478 (463.89, -637.4911) -> (463.89, -640.4911)
  line L1479 (463.89, -640.4911) -> (472.6177, -640.4911)
  line L1480 (472.6177, -181.4314) -> (472.6177, -178.4314)
  line L1481 (481.2233, -181.4314) -> (472.6177, -181.4314)
  line L1482 (472.6177, -640.4911) -> (472.6177, -637.4911)
  line L1483 (472.6177, -637.4911) -> (481.2233, -637.4911)
  line L1484 (481.2233, -178.4314) -> (481.2233, -181.4314)
  line L1485 (489.951, -178.4314) -> (481.2233, -178.4314)
  line L1486 (481.2233, -637.4911) -> (481.2233, -640.4911)
  line L1487 (481.2233, -640.4911) -> (489.951, -640.4911)
  line L1488 (489.951, -181.4314) -> (489.951, -178.4314)
  line L1489 (498.5563, -181.4314) -> (489.9507, -181.4314)
  line L1490 (489.951, -640.4911) -> (489.951, -637.4911)
  line L1491 (489.951, -637.4911) -> (498.5563, -637.4911)
  line L1492 (498.5563, -178.4314) -> (498.5563, -181.4314)
  line L1493 (507.2844, -178.4314) -> (498.5563, -178.4314)
  line L1494 (507.2844, -640.4911) -> (498.5563, -640.4911)
  line L1495 (498.5563, -640.4911) -> (498.5563, -637.4911)
  line L1496 (507.2844, -181.4314) -> (507.2844, -178.4314)
  line L1497 (515.89, -181.4314) -> (507.2844, -181.4314)
  line L1498 (507.2844, -640.4911) -> (507.2844, -637.4911)
  line L1499 (507.2844, -637.4911) -> (515.89, -637.4911)
  line L1500 (515.89, -178.4314) -> (515.89, -181.4314)
  line L1501 (524.6173, -178.4314) -> (515.89, -178.4314)
  line L1502 (515.89, -637.4911) -> (515.89, -640.4911)
  line L1503 (515.89, -640.4911) -> (524.6173, -640.4911)
  line L1504 (524.6173, -181.4314) -> (524.6173, -178.4314)
  line L1505 (533.2233, -181.4314) -> (524.617, -181.4314)
  line L1506 (524.6173, -640.4911) -> (524.6173, -637.4911)
  line L1507 (524.6173, -637.4911) -> (533.2233, -637.4911)
  line L1508 (533.2233, -178.4314) -> (533.2233, -181.4314)
  line L1509 (541.9507, -178.4314) -> (533.2233, -178.4314)
  line L1510 (533.2233, -637.4911) -> (533.2233, -640.4911)
  line L1511 (533.2233, -640.4911) -> (541.9507, -640.4911)
  line L1512 (541.9507, -181.4314) -> (541.9507, -178.4314)
  line L1513 (550.5567, -181.4314) -> (541.9507, -181.4314)
  line L1514 (541.9507, -640.4911) -> (541.9507, -637.4911)
  line L1515 (541.9507, -637.4911) -> (550.5567, -637.4911)
  line L1516 (550.5567, -178.4314) -> (550.5567, -181.4314)
  line L1517 (559.284, -178.4314) -> (550.5567, -178.4314)
  line L1518 (550.5567, -637.4911) -> (550.5567, -640.4911)
  line L1519 (550.5567, -640.4911) -> (559.284, -640.4911)
  line L1520 (559.284, -181.4314) -> (559.284, -178.4314)
  line L1521 (567.89, -181.4314) -> (559.2837, -181.4314)
  line L1522 (559.284, -640.4911) -> (559.284, -637.4911)
  line L1523 (559.284, -637.4911) -> (567.89, -637.4911)
  line L1524 (567.89, -178.4314) -> (567.89, -181.4314)
  line L1525 (576.6174, -178.4314) -> (567.89, -178.4314)
  line L1526 (567.89, -637.4911) -> (567.89, -640.4911)
  line L1527 (567.89, -640.4911) -> (576.6174, -640.4911)
  line L1528 (576.6174, -181.4314) -> (576.6174, -178.4314)
  line L1529 (585.223, -181.4314) -> (576.6174, -181.4314)
  line L1530 (576.6174, -640.4911) -> (576.6174, -637.4911)
  line L1531 (576.6174, -637.4911) -> (585.223, -637.4911)
  line L1532 (585.223, -178.4314) -> (585.223, -181.4314)
  line L1533 (593.9507, -178.4314) -> (585.223, -178.4314)
  line L1534 (585.223, -637.4911) -> (585.223, -640.4911)
  line L1535 (585.223, -640.4911) -> (593.9507, -640.4911)
  line L1536 (593.9507, -181.4314) -> (593.9507, -178.4314)
  line L1537 (602.5563, -181.4314) -> (593.9504, -181.4314)
  line L1538 (593.9507, -640.4911) -> (593.9507, -637.4911)
  line L1539 (593.9507, -637.4911) -> (602.5563, -637.4911)
  line L1540 (602.5563, -178.4314) -> (602.5563, -181.4314)
  line L1541 (611.2837, -178.4314) -> (602.5563, -178.4314)
  line L1542 (602.5563, -637.4911) -> (602.5563, -640.4911)
  line L1543 (602.5563, -640.4911) -> (611.2837, -640.4911)
  line L1544 (611.2837, -181.4314) -> (611.2837, -178.4314)
  line L1545 (619.8897, -181.4314) -> (611.2837, -181.4314)
  line L1546 (611.2837, -640.4911) -> (611.2837, -637.4911)
  line L1547 (611.2837, -637.4911) -> (619.8897, -637.4911)
  line L1548 (619.8897, -178.4314) -> (619.8897, -181.4314)
  line L1549 (628.6174, -178.4314) -> (619.8897, -178.4314)
  line L1550 (619.8897, -637.4911) -> (619.8897, -640.4911)
  line L1551 (619.8897, -640.4911) -> (628.6174, -640.4911)
  line L1552 (628.6174, -181.4314) -> (628.6174, -178.4314)
  line L1553 (637.223, -181.4314) -> (628.6174, -181.4314)
  line L1554 (628.6174, -640.4911) -> (628.6174, -637.4911)
  line L1555 (628.6174, -637.4911) -> (637.223, -637.4911)
  line L1556 (637.223, -178.4314) -> (637.223, -181.4314)
  line L1557 (645.9507, -178.4314) -> (637.223, -178.4314)
  line L1558 (637.223, -637.4911) -> (637.223, -640.4911)
  line L1559 (637.223, -640.4911) -> (645.9507, -640.4911)
  line L1560 (645.9507, -181.4314) -> (645.9507, -178.4314)
  line L1561 (654.556, -181.4314) -> (645.9504, -181.4314)
  line L1562 (645.9507, -640.4911) -> (645.9507, -637.4911)
  line L1563 (645.9507, -637.4911) -> (654.556, -637.4911)
  line L1564 (654.556, -178.4314) -> (654.556, -181.4314)
  line L1565 (663.2841, -178.4314) -> (654.556, -178.4314)
  line L1566 (654.556, -637.4911) -> (654.556, -640.4911)
  line L1567 (654.556, -640.4911) -> (663.2841, -640.4911)
  line L1568 (663.2841, -181.4314) -> (663.2841, -178.4314)
  line L1569 (671.8894, -181.4314) -> (663.2841, -181.4314)
  line L1570 (663.2841, -640.4911) -> (663.2841, -637.4911)
  line L1571 (663.2841, -637.4911) -> (671.8894, -637.4911)
  line L1572 (671.8894, -178.4314) -> (671.8894, -181.4314)
  line L1573 (680.6171, -178.4314) -> (671.8894, -178.4314)
  line L1574 (671.8894, -637.4911) -> (671.8894, -640.4911)
  line L1575 (671.8894, -640.4911) -> (680.6171, -640.4911)
  line L1576 (680.6171, -181.4314) -> (680.6171, -178.4314)
  line L1577 (689.2227, -181.4314) -> (680.6171, -181.4314)
  line L1578 (680.6171, -640.4911) -> (680.6171, -637.4911)
  line L1579 (680.6171, -637.4911) -> (689.2227, -637.4911)
  line L1580 (689.2227, -178.4314) -> (689.2227, -181.4314)
  line L1581 (697.9504, -178.4314) -> (689.2227, -178.4314)
  line L1582 (689.2227, -637.4911) -> (689.2227, -640.4911)
  line L1583 (689.2227, -640.4911) -> (697.9504, -640.4911)
  line L1584 (697.9504, -181.4314) -> (697.9504, -178.4314)
  line L1585 (706.556, -181.4314) -> (697.9504, -181.4314)
  line L1586 (697.9504, -640.4911) -> (697.9504, -637.4911)
  line L1587 (697.9504, -637.4911) -> (706.556, -637.4911)
  line L1588 (706.556, -178.4314) -> (706.556, -181.4314)
  line L1589 (715.2837, -178.4314) -> (706.556, -178.4314)
  line L1590 (706.556, -637.4911) -> (706.556, -640.4911)
  line L1591 (706.556, -640.4911) -> (715.2837, -640.4911)
  line L1592 (715.2837, -181.4314) -> (715.2837, -178.4314)
  line L1593 (723.8894, -181.4314) -> (715.2834, -181.4314)
  line L1594 (715.2837, -640.4911) -> (715.2837, -637.4911)
  line L1595 (715.2837, -637.4911) -> (723.8894, -637.4911)
  line L1596 (723.8894, -178.4314) -> (723.8894, -181.4314)
  line L1597 (732.6171, -178.4314) -> (723.8894, -178.4314)
  line L1598 (723.8894, -637.4911) -> (723.8894, -640.4911)
  line L1599 (723.8894, -640.4911) -> (732.6171, -640.4911)
  line L1600 (732.6171, -181.4314) -> (732.6171, -178.4314)
  line L1601 (732.6171, -637.4911) -> (741.2834, -637.4911)
  line L1602 (741.2834, -181.4314) -> (732.6171, -181.4314)
  line L1603 (732.6171, -640.4911) -> (732.6171, -637.4911)
  line L1604 (741.2834, -637.4911) -> (741.2834, -628.8873)
  line L1605 (741.2834, -628.8876) -> (744.2834, -628.8876)
  line L1606 (741.2834, -620.2227) -> (741.2834, -611.6799)
  line L1607 (744.2834, -620.2227) -> (741.2834, -620.2227)
  line L1608 (741.2834, -611.6799) -> (744.2834, -611.6799)
  line L1609 (741.2834, -603.0153) -> (741.2834, -594.4725)
  line L1610 (744.2834, -603.0153) -> (741.2834, -603.0153)
  line L1611 (741.2834, -594.4725) -> (744.2834, -594.4725)
  line L1612 (741.2834, -585.8079) -> (741.2834, -577.2651)
  line L1613 (744.2834, -585.8079) -> (741.2834, -585.8079)
  line L1614 (741.2834, -577.2651) -> (744.2834, -577.2651)
  line L1615 (741.2834, -568.6002) -> (741.2834, -560.0573)
  line L1616 (744.2834, -568.6002) -> (741.2834, -568.6002)
  line L1617 (741.2834, -560.0573) -> (744.2834, -560.0573)
  line L1618 (741.2834, -551.3928) -> (741.2834, -542.8499)
  line L1619 (744.2834, -551.3928) -> (741.2834, -551.3928)
  line L1620 (741.2834, -542.8499) -> (744.2834, -542.8499)
  line L1621 (741.2834, -534.185) -> (741.2834, -525.6425)
  line L1622 (744.2834, -534.185) -> (741.2834, -534.185)
  line L1623 (741.2834, -525.6425) -> (744.2834, -525.6425)
  line L1624 (741.2834, -516.9776) -> (741.2834, -508.4348)
  line L1625 (744.2834, -516.9776) -> (741.2834, -516.9776)
  line L1626 (741.2834, -508.4348) -> (744.2834, -508.4348)
  line L1627 (741.2834, -499.7702) -> (741.2834, -491.2274)
  line L1628 (744.2834, -499.7702) -> (741.2834, -499.7702)
  line L1629 (741.2834, -491.2274) -> (744.2834, -491.2274)
  line L1630 (741.2834, -482.5625) -> (741.2834, -474.02)
  line L1631 (744.2834, -482.5625) -> (741.2834, -482.5625)
  line L1632 (741.2834, -474.02) -> (744.2834, -474.02)
  line L1633 (741.2834, -465.3551) -> (741.2834, -456.8122)
  line L1634 (744.2834, -465.3551) -> (741.2834, -465.3551)
  line L1635 (741.2834, -456.8122) -> (744.2834, -456.8122)
  line L1636 (741.2834, -448.1477) -> (741.2834, -439.6048)
  line L1637 (744.2834, -448.1477) -> (741.2834, -448.1477)
  line L1638 (741.2834, -439.6048) -> (744.2834, -439.6048)
  line L1639 (741.2834, -430.9403) -> (741.2834, -422.3974)
  line L1640 (744.2834, -430.9403) -> (741.2834, -430.9403)
  line L1641 (741.2834, -422.3974) -> (744.2834, -422.3974)
  line L1642 (741.2834, -413.7329) -> (741.2834, -405.1897)
  line L1643 (744.2834, -413.7329) -> (741.2834, -413.7329)
  line L1644 (741.2834, -405.1897) -> (744.2834, -405.1897)
  line L1645 (741.2834, -396.5255) -> (741.2834, -387.9823)
  line L1646 (744.2834, -396.5255) -> (741.2834, -396.5255)
  line L1647 (741.2834, -387.9826) -> (744.2834, -387.9826)
  line L1648 (741.2834, -379.3177) -> (741.2834, -370.7749)
  line L1649 (744.2834, -379.3177) -> (741.2834, -379.3177)
  line L1650 (741.2834, -370.7752) -> (744.2834, -370.7752)
  line L1651 (741.2834, -362.1103) -> (741.2834, -353.5675)
  line L1652 (744.2834, -362.1103) -> (741.2834, -362.1103)
  line L1653 (741.2834, -353.5675) -> (744.2834, -353.5675)
  line L1654 (741.2834, -344.9029) -> (741.2834, -336.3597)
  line L1655 (744.2834, -344.9029) -> (741.2834, -344.9029)
  line L1656 (741.2834, -336.3601) -> (744.2834, -336.3601)
  line L1657 (741.2834, -327.6952) -> (741.2834, -319.1523)
  line L1658 (744.2834, -327.6952) -> (741.2834, -327.6952)
  line L1659 (741.2834, -319.1527) -> (744.2834, -319.1527)
  line L1660 (741.2834, -310.4878) -> (741.2834, -301.9449)
  line L1661 (744.2834, -310.4878) -> (741.2834, -310.4878)
  line L1662 (741.2834, -301.9449) -> (744.2834, -301.9449)
  line L1663 (741.2834, -293.2804) -> (741.2834, -284.7372)
  line L1664 (744.2834, -293.2804) -> (741.2834, -293.2804)
  line L1665 (741.2834, -284.7375) -> (744.2834, -284.7375)
  line L1666 (741.2834, -276.0726) -> (741.2834, -267.5298)
  line L1667 (744.2834, -276.0726) -> (741.2834, -276.0726)
  line L1668 (741.2834, -267.5298) -> (744.2834, -267.5298)
  line L1669 (741.2834, -258.8652) -> (741.2834, -250.3224)
  line L1670 (744.2834, -258.8652) -> (741.2834, -258.8652)
  line L1671 (741.2834, -250.3224) -> (744.2834, -250.3224)
  line L1672 (741.2834, -241.6578) -> (741.2834, -233.1146)
  line L1673 (744.2834, -241.6578) -> (741.2834, -241.6578)
  line L1674 (741.2834, -233.115) -> (744.2834, -233.115)
  line L1675 (741.2834, -224.4501) -> (741.2834, -215.9072)
  line L1676 (744.2834, -224.4501) -> (741.2834, -224.4501)
  line L1677 (741.2834, -215.9072) -> (744.2834, -215.9072)
  line L1678 (741.2834, -207.2427) -> (741.2834, -198.6998)
  line L1679 (744.2834, -207.2427) -> (741.2834, -207.2427)
  line L1680 (741.2834, -198.6998) -> (744.2834, -198.6998)
  line L1681 (741.2834, -190.0353) -> (741.2834, -181.431)
  line L1682 (744.2834, -190.0353) -> (741.2834, -190.0353)
  line L1683 (744.2834, -628.8876) -> (744.2834, -620.2224)
  line L1684 (744.2834, -611.6799) -> (744.2834, -603.015)
  line L1685 (744.2834, -594.4725) -> (744.2834, -585.8076)
  line L1686 (744.2834, -577.2651) -> (744.2834, -568.5998)
  line L1687 (744.2834, -560.0573) -> (744.2834, -551.3924)
  line L1688 (744.2834, -542.8499) -> (744.2834, -534.185)
  line L1689 (744.2834, -525.6425) -> (744.2834, -516.9773)
  line L1690 (744.2834, -508.4348) -> (744.2834, -499.7699)
  line L1691 (744.2834, -491.2274) -> (744.2834, -482.5621)
  line L1692 (744.2834, -474.02) -> (744.2834, -465.3547)
  line L1693 (744.2834, -456.8122) -> (744.2834, -448.1473)
  line L1694 (744.2834, -439.6048) -> (744.2834, -430.9399)
  line L1695 (744.2834, -422.3974) -> (744.2834, -413.7325)
  line L1696 (744.2834, -405.1897) -> (744.2834, -396.5251)
  line L1697 (744.2834, -387.9826) -> (744.2834, -379.3177)
  line L1698 (744.2834, -370.7752) -> (744.2834, -362.1103)
  line L1699 (744.2834, -353.5675) -> (744.2834, -344.9026)
  line L1700 (744.2834, -336.3601) -> (744.2834, -327.6952)
  line L1701 (744.2834, -319.1527) -> (744.2834, -310.4878)
  line L1702 (744.2834, -301.9449) -> (744.2834, -293.28)
  line L1703 (744.2834, -284.7375) -> (744.2834, -276.0726)
  line L1704 (744.2834, -267.5298) -> (744.2834, -258.8649)
  line L1705 (744.2834, -250.3224) -> (744.2834, -241.6575)
  line L1706 (744.2834, -233.115) -> (744.2834, -224.4501)